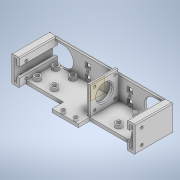
# Autodesk Inventor part: xStart
Saved by Autodesk Inventor 2022 (Build 260153000, 153)
## iProperties
Created: 2020-01-24
Part Number: xStart
Material: Generic
Document SubType Name: Modeling
Designer: PAB
Density: 1 g/cm^3
Appearance: Default
Author: PAB
Autodesk Inventor part; units mm, degrees
ref_plane "YZ Plane" through (0, 0, 0) normal (1, 0, 0) x (0, 1, 0)
ref_plane "XZ Plane" through (0, 0, 0) normal (0, 1, 0) x (-1, 0, 0)
ref_plane "XY Plane" through (0, 0, 0) normal (0, 0, 1) x (1, 0, 0)
sketch "Sketch1" plane through (0, 0, 0) normal (0, 1, 0) x (-1, 0, 0)
  line L0 (94, 24) -> (-94, 24)
  line L1 (-94, 24) -> (-94, -24)
  line L2 (-94, -24) -> (94, -24)
  line L3 (94, -24) -> (94, 24)
  point P0 (0, 0)
  dimension "d0" = 188
  dimension "d1" = 48
  constraints: 8 end point, 2 parallel, 1 horizontal, 1 perpendicular
  measures "d0" distance of L2.end L1.end
  measures "d1" distance of L1.end L0.end
extrude "Extrusion1" add sketch "Sketch1" along normal blind 5
sketch "Sketch2" plane through (0, 5, 0) normal (0, 1, 0) x (1, 0, 0)
  line L0 (-94, 24) -> (-94, -24) projected
  line L1 (94, 24) -> (-94, 24) projected
  line L2 (-94, -24) -> (-90, -24)
  line L3 (-90, -24) -> (-90, 24)
  line L4 (-90, 24) -> (-94, 24)
  line L5 (-94, 24) -> (-94, -24)
  line L6 (94, -24) -> (94, 24) projected
  line L7 (-90, 24) -> (94, 24)
  line L8 (94, 24) -> (94, 20)
  line L9 (94, 20) -> (-90, 20)
  line L10 (-90, 20) -> (-90, 24)
  line L11 (-94, -24) -> (94, -24) projected
  line L12 (94, 20) -> (90, 20)
  line L13 (90, 20) -> (90, -24)
  line L14 (90, -24) -> (94, -24)
  line L15 (94, -24) -> (94, 20)
  point P0 (0, 0)
  point P1 (-90, 20)
  dimension "d4" = 4
  dimension "d5" = 4
  dimension "d6" = 4
  constraints: 24 end point, 6 parallel, 3 horizontal, 3 perpendicular, 3 point on line
  measures "d4" distance of L4.end L3.end
  measures "d5" distance of L7.end L8.end
  measures "d6" distance of L14.end L13.end
extrude "Extrusion2" add sketch "Sketch2" along normal blind 35 contours L1 L3 L2 L0 | L1 L6 L9 L3 | L13 L9 L6 L11
sketch "Sketch3" plane through (-90, 5, 24) normal (1, 0, 0) x (0, 0, -1)
  line L0 (0, 0) -> (0, 35) projected
  line L1 (44, 0) -> (44, 35) projected
  line L2 (0, 35) -> (44, 35)
  line L3 (44, 35) -> (44, 31)
  line L4 (44, 31) -> (0, 31)
  line L5 (0, 31) -> (0, 35)
  point P0 (24, -5)
  dimension "d9" = 4
  constraints: 8 end point, 2 parallel, 1 horizontal, 1 perpendicular, 1 point on line
  measures "d9" distance of L2.end L3.end
extrude "Extrusion3" add sketch "Sketch3" along normal blind 8
sketch "Sketch4" plane through (0, 5, 0) normal (0, 1, 0) x (1, 0, 0)
  line L0 (90, 20) -> (-90, 20) projected
  line L1 (-82, -24) -> (-86, -24)
  line L2 (-86, -24) -> (-86, 20)
  line L3 (-86, 20) -> (-82, 20)
  line L4 (-82, 20) -> (-82, -24)
  point P0 (0, 0)
  dimension "d12" = 4
  constraints: 8 end point, 2 parallel, 1 horizontal, 1 perpendicular, 1 point on line
  measures "d12" distance of L2.end L3.end
extrude "Extrusion4" add sketch "Sketch4" along normal blind 8
sketch "Sketch5" plane through (-90, 36, -20) normal (0, -1, 0) x (1, 0, 0)
  line L0 (0, 44) -> (8, 44) projected
  line L1 (8, 44) -> (8, 0) projected
  line L2 (4, 44) -> (8, 44)
  line L3 (8, 44) -> (8, 0)
  line L4 (8, 0) -> (4, 0)
  line L5 (4, 0) -> (4, 44)
  point P0 (90, 20)
  constraints: 8 end point, 2 parallel, 1 horizontal, 1 midpoint, 1 perpendicular
extrude "Extrusion5" add sketch "Sketch5" along normal blind 8
sketch "Sketch6" plane through (90, 5, -20) normal (0, 0, 1) x (1, 0, 0)
  line L0 (-180, 31) -> (-176, 31) projected
  line L1 (-176, 0) -> (-176, 8) projected
  line L2 (-180, 31) -> (-176, 31)
  line L3 (-176, 31) -> (-176, 0)
  line L4 (-176, 0) -> (-180, 0)
  line L5 (-180, 0) -> (-180, 31)
  line L6 (-172, 23) -> (-176, 23) projected
  line L7 (-176, 8) -> (-172, 8) projected
  line L8 (-176, 23) -> (-172, 23)
  line L9 (-172, 23) -> (-172, 8)
  line L10 (-172, 8) -> (-176, 8)
  line L11 (-176, 8) -> (-176, 23)
  line L12 (-172, 35) -> (-172, 23) projected
  line L13 (-172, 0) -> (0, 0) projected
  line L14 (-172, 31) -> (-159.5, 31)
  line L15 (-159.5, 31) -> (-159.5, 0)
  line L16 (-159.5, 0) -> (-172, 0)
  line L17 (-172, 0) -> (-172, 31)
  arc A0 (-159.5, 0) -> (-159.5, 31) centre (-159.5, 15.5) ccw
  point P0 (-90, -5)
  point P1 (-172, 8)
  dimension "d17" = 12.5
  dimension "d18" = 15.5
  constraints: 24 end point, 6 parallel, 3 horizontal, 3 perpendicular, 3 point on line, 2 point on circle, 1 centre point
  measures "d17" distance of L15.end L16.end
  measures "d18" radius of A0
extrude "Extrusion6" cut sketch "Sketch6" against normal blind 8
sketch "Sketch7" plane through (-94, 0, 24) normal (0, 0, 1) x (1, 0, 0)
  line L0 (12, 36) -> (12, 28) projected
  line L1 (0, 40) -> (12, 40) projected
  line L2 (12, 28) -> (8, 28)
  line L3 (8, 28) -> (8, 40)
  line L4 (8, 40) -> (12, 40)
  line L5 (12, 40) -> (12, 28)
  line L6 (8, 13) -> (12, 13) projected
  line L7 (188, 0) -> (0, 0) projected
  line L8 (12, 13) -> (8, 13)
  line L9 (8, 13) -> (8, 0)
  line L10 (8, 0) -> (12, 0)
  line L11 (12, 0) -> (12, 13)
  line L12 (8, 0) -> (0, 0)
  line L13 (0, 0) -> (0, 5)
  line L14 (0, 5) -> (8, 5)
  line L15 (8, 5) -> (8, 0)
  line L16 (0, 5) -> (4, 5)
  line L17 (4, 5) -> (4, 40)
  line L18 (4, 40) -> (0, 40)
  line L19 (0, 40) -> (0, 5)
  line L20 (8, 36) -> (4, 36) projected
  line L21 (4, 40) -> (8, 40)
  line L22 (8, 40) -> (8, 36)
  line L23 (8, 36) -> (4, 36)
  line L24 (4, 36) -> (4, 40)
  point P0 (94, 0)
  point P1 (8, 13)
  point P2 (8, 5)
  dimension "d21" = 4
  dimension "d22" = 4
  dimension "d103" = 5
  constraints: 40 end point, 10 parallel, 5 horizontal, 5 perpendicular, 3 point on line
  measures "d21" distance of L3.end L4.end
  measures "d22" distance of L10.end L9.end
  measures "d103" distance between parallel lines of L7 L14
extrude "Extrusion7" add sketch "Sketch7" along normal blind 10
sketch "Sketch8" plane through (0, 5, 0) normal (0, 1, 0) x (1, 0, 0)
  point P0 (0, 0)
sketch "Sketch9" plane through (0, 5, 0) normal (0, 1, 0) x (1, 0, 0)
  circle A0 centre (-75, -14) radius 3
  circle A1 centre (-75, 14) radius 3
  circle A2 centre (-49, -14) radius 3
  circle A3 centre (-49, 14) radius 3
  point P0 (0, 0)
  dimension "d25" = 6
  dimension "d26" = 6
  dimension "d27" = 6
  dimension "d28" = 6
  constraints: 4 centre point
  measures "d25" diameter of A0
  measures "d26" diameter of A1
  measures "d27" diameter of A2
  measures "d28" diameter of A3
extrude "Extrusion8" cut sketch "Sketch9" against normal blind 10
sketch "Sketch10" plane through (0, 5, 0) normal (0, 1, 0) x (1, 0, 0)
  line L0 (-82, 20) -> (90, 20) projected
  line L1 (-82, -24) -> (94, -24) projected
  line L2 (15, 20) -> (10, 20)
  line L3 (10, 20) -> (10, -24)
  line L4 (10, -24) -> (15, -24)
  line L5 (15, -24) -> (15, 20)
  line L6 (90, 20) -> (90, -24) projected
  point P0 (0, 0)
  dimension "d31" = 5
  dimension "d32" = 75
  constraints: 8 end point, 2 parallel, 2 point on line, 1 horizontal, 1 perpendicular
  measures "d31" distance of L4.end L3.end
  measures "d32" distance between parallel lines of L6 L5
extrude "Extrusion9" add sketch "Sketch10" along normal blind 42.3 contours L0 L5 L1 L3
sketch "Sketch11" plane through (15, 5, 24) normal (1, 0, 0) x (0, 0, -1)
  circle A0 centre (38.35, 5.65) radius 2
  circle A1 centre (38.35, 36.65) radius 2
  circle A2 centre (7.35, 5.65) radius 2
  circle A3 centre (7.35, 36.65) radius 2
  circle A4 centre (22.85, 21.15) radius 12.5
  line L0 (44, 35) -> (44, 42.3) projected
  line L1 (44, 0) -> (0, 0) projected
  point P0 (24, -5)
  dimension "d35" = 4
  dimension "d36" = 4
  dimension "d37" = 4
  dimension "d38" = 4
  dimension "d39" = 25
  dimension "d98" = 36.65
  dimension "d99" = 5.65
  dimension "d100" = 5.65
  dimension "d101" = 36.65
  dimension "d102" = 21.15
  dimension "d104" = 5.65
  dimension "d105" = 5.65
  dimension "d106" = 21.15
  dimension "d107" = 36.65
  dimension "d108" = 36.65
  constraints: 5 centre point
  measures "d35" diameter of A0
  measures "d36" diameter of A1
  measures "d37" diameter of A2
  measures "d38" diameter of A3
  measures "d39" diameter of A4
  measures "d98" distance from line of L0 A3.centre
  measures "d99" distance from line of L0 A1.centre
  measures "d100" distance from line of L0 A0.centre
  measures "d101" distance from line of L0 A2.centre
  measures "d102" distance from line of L0 A4.centre
  measures "d104" distance from line of L1 A0.centre
  measures "d105" distance from line of L1 A2.centre
  measures "d106" distance from line of L1 A4.centre
  measures "d107" distance from line of L1 A3.centre
  measures "d108" distance from line of L1 A1.centre
extrude "Extrusion10" cut sketch "Sketch11" against normal blind 42.3
sketch "Sketch12" plane through (0, 5, 0) normal (0, 1, 0) x (1, 0, 0)
  point P0 (0, 0)
sketch "Sketch13" plane through (-82, 5, 24) normal (0, 0, 1) x (1, 0, 0)
  point P0 (82, -5)
sketch "Sketch17" plane through (0, 5, 0) normal (0, 1, 0) x (1, 0, 0)
  circle A0 centre (-75, -14) radius 3 projected
  circle A1 centre (-75, -14) radius 5
  circle A2 centre (-75, 14) radius 3 projected
  circle A3 centre (-75, 14) radius 5
  circle A4 centre (-49, 14) radius 3 projected
  circle A5 centre (-49, 14) radius 5
  circle A6 centre (-49, -14) radius 3 projected
  circle A7 centre (-49, -14) radius 5
  point P0 (0, 0)
  dimension "d54" = 10
  dimension "d55" = 10
  dimension "d56" = 10
  dimension "d57" = 10
  constraints: 4 centre point, 4 coincident
  measures "d54" diameter of A1
  measures "d55" diameter of A3
  measures "d56" diameter of A5
  measures "d57" diameter of A7
extrude "Extrusion14" add sketch "Sketch17" along normal blind 5
mirror "Mirror2" about plane through (0, 0, 0) normal (1, 0, 0) of "Extrusion14", "Extrusion8", "Extrusion7", "Extrusion6", "Extrusion5", "Extrusion4", "Extrusion3"
sketch "Sketch18" plane through (-82, 5, 24) normal (0, 0, 1) x (1, 0, 0)
  line L0 (97, 0) -> (97, 42.3) projected
  line L1 (97, 0) -> (57, 0)
  line L2 (57, 0) -> (57, -5)
  line L3 (57, -5) -> (97, -5)
  line L4 (97, -5) -> (97, 0)
  point P0 (82, -5)
  dimension "d60" = 40
  dimension "d61" = 5
  constraints: 8 end point, 2 parallel, 1 horizontal, 1 perpendicular
  measures "d60" distance of L3.end L2.end
  measures "d61" distance of L2.end L1.end
extrude "Extrusion15" add sketch "Sketch18" along normal blind 17.5
sketch "Sketch19" plane through (0, 5, 0) normal (0, 1, 0) x (1, 0, 0)
  circle A0 centre (-11, -38.5) radius 2
  circle A1 centre (8, -38.5) radius 2
  point P0 (0, 0)
  dimension "d64" = 4
  dimension "d65" = 4
  constraints: 2 centre point
  measures "d64" diameter of A0
  measures "d65" diameter of A1
extrude "Extrusion16" cut sketch "Sketch19" against normal blind 17.5
sketch "Sketch20" plane through (0, 5, 0) normal (0, 1, 0) x (1, 0, 0)
  circle A0 centre (-11, -38.5) radius 2 projected
  circle A1 centre (-11, -38.5) radius 3
  circle A2 centre (8, -38.5) radius 2 projected
  circle A3 centre (8, -38.5) radius 3
  point P0 (0, 0)
  dimension "d68" = 6
  dimension "d69" = 6
  constraints: 2 centre point, 2 coincident
  measures "d68" diameter of A1
  measures "d69" diameter of A3
extrude "Extrusion17" add sketch "Sketch20" along normal blind 4
sketch "Sketch21" plane through (94, 0, -24) normal (1, 0, 0) x (0, 0, -1)
  circle A0 centre (-48, 31) radius 2
  circle A1 centre (-48, 8) radius 2
  line L0 (-58, 40) -> (-58, 0) projected
  point P0 (-24, 0)
  dimension "d72" = 4
  dimension "d73" = 4
  dimension "d74" = 10
  dimension "d75" = 10
  constraints: 2 centre point
  measures "d72" diameter of A0
  measures "d73" diameter of A1
  measures "d74" distance from line of L0 A0.centre
  measures "d75" distance from line of L0 A1.centre
extrude "Extrusion18" cut sketch "Sketch21" against normal blind 20
mirror "Mirror3" about plane through (0, 0, 0) normal (1, 0, 0) of "Extrusion18"
sketch "Sketch22" plane through (94, 0, -24) normal (0, 0, -1) x (-1, 0, 0)
  line L0 (122, 31) -> (130, 31)
  line L1 (130, 31) -> (130, 23)
  line L2 (130, 23) -> (122, 23)
  line L3 (122, 23) -> (122, 31)
  line L4 (122, 15) -> (130, 15)
  line L5 (130, 15) -> (130, 7)
  line L6 (130, 7) -> (122, 7)
  line L7 (122, 7) -> (122, 15)
  circle A0 centre (126, 19) radius 2
  point P0 (94, 0)
  dimension "d78" = 8
  dimension "d79" = 8
  dimension "d80" = 8
  dimension "d81" = 8
  dimension "d82" = 4
  constraints: 16 end point, 4 parallel, 2 horizontal, 2 perpendicular, 1 centre point, 1 point on line
  measures "d78" distance of L1.end L2.end
  measures "d79" distance of L0.end L1.end
  measures "d80" distance of L5.end L6.end
  measures "d81" distance of L4.end L5.end
  measures "d82" diameter of A0
extrude "Extrusion19" cut sketch "Sketch22" against normal blind 20
mirror "Mirror4" about plane through (0, 0, 0) normal (1, 0, 0) of "Extrusion19"
fillet "Fillet1" radius 1.5 28 edges at (0, 40, -24) (94, 40, 5) (-94, 40, 5) (94, 20, -24) (-94, 20, -24) (82, 40, 7) (-82, 40, 7) (-82, 0, 29) (82, 0, 29) (-94, 0, 5) (94, 0, 5) (0, 0, -24) (-36, 40, -20) (48.5, 40, -20) (15, 47.3, 2) (10, 47.3, 2) (15, 43.65, -20) (10, 43.65, -20) (12.5, 47.3, -20) (15, 26.15, 24) (10, 26.15, 24) (75.75, 5, -24) (75.75, 36, -24) (54, 20.5, -24) (-75.75, 36, -24) (-75.75, 5, -24) (-54, 20.5, -24) (15, 26.15, 13.65)
ref_plane "Work Plane1" through (19, 40.65, 16.65) normal (1, 0, 0) x (0, 0, -1)
sketch "Sketch24" plane through (19, 40.65, 16.65) normal (1, 0, 0) x (0, 0, -1)
  circle A0 centre (0, 0) radius 3
  circle A1 centre (31, 0) radius 2 projected
  circle A2 centre (31, 0) radius 3
  circle A3 centre (31, -31) radius 4 projected
  circle A4 centre (31, -31) radius 3
  circle A5 centre (0, -31) radius 2 projected
  circle A6 centre (0, -31) radius 3
  point P0 (16.65, -40.65)
  dimension "d92" = 6
  dimension "d93" = 6
  dimension "d94" = 6
  dimension "d95" = 6
  constraints: 4 centre point, 3 coincident
  measures "d92" diameter of A0
  measures "d93" diameter of A2
  measures "d94" diameter of A4
  measures "d95" diameter of A6
extrude "Extrusion21" cut sketch "Sketch24" against normal blind 3 contours A0 | A1 | A2 | A4 | A5 | A6
body "Solid1"
